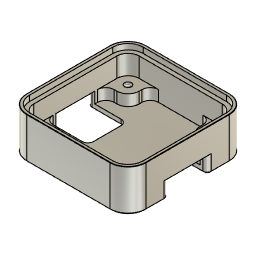
simplest_knob_case_tutorial (Autodesk Fusion 360 design; units mm, degrees)
Autodesk Fusion 360 part; units mm, degrees
sketch "sketch_for_main_body_shape" plane through (0, 0, 0) normal (0, 0, 1) x (1, 0, 0)
  line L0 (15, -18.5) -> (-15, -18.5) construction
  line L1 (-18.5, -15) -> (-18.5, 15) construction
  line L2 (-15, 18.5) -> (15, 18.5) construction
  line L3 (18.5, 15) -> (18.5, -15) construction
  line L4 (18.5, -18.5) -> (-18.5, 18.5) construction
  line L5 (-18.5, -18.5) -> (18.5, 18.5) construction
  arc A0 (-15, 18.5) -> (-18.5, 15) centre (-15, 15) ccw construction
  arc A1 (-18.5, -15) -> (-15, -18.5) centre (-15, -15) ccw construction
  arc A2 (15, -18.5) -> (18.5, -15) centre (15, -15) ccw construction
  arc A3 (18.5, 15) -> (15, 18.5) centre (15, 15) ccw construction
  arc A4 (19, 15) -> (15, 19) centre (15, 15) ccw
  line L6 (-15, 19) -> (15, 19)
  arc A5 (-15, 19) -> (-19, 15) centre (-15, 15) ccw
  line L7 (-19, -15) -> (-19, 15)
  arc A6 (-19, -15) -> (-15, -19) centre (-15, -15) ccw
  line L8 (15, -19) -> (-15, -19)
  arc A7 (15, -19) -> (19, -15) centre (15, -15) ccw
  line L9 (19, 15) -> (19, -15)
  arc A8 (21.5, 15) -> (15, 21.5) centre (15, 15) ccw
  line L10 (-15, 21.5) -> (15, 21.5)
  arc A9 (-15, 21.5) -> (-21.5, 15) centre (-15, 15) ccw
  line L11 (-21.5, -15) -> (-21.5, 15)
  arc A10 (-21.5, -15) -> (-15, -21.5) centre (-15, -15) ccw
  line L12 (15, -21.5) -> (-15, -21.5)
  arc A11 (15, -21.5) -> (21.5, -15) centre (15, -15) ccw
  line L13 (21.5, 15) -> (21.5, -15)
  circle A12 centre (-15, 15) radius 4
  line L14 (-11, 15) -> (-11, 19)
  line L15 (-15, 11) -> (-19, 11)
  circle A13 centre (15, 15) radius 4
  line L16 (11, 15) -> (11, 19)
  line L17 (15, 11) -> (19, 11)
  line L18 (-37.3211, 0) -> (37.3211, 0) construction
  line L19 (-11, -15) -> (-11, -19)
  circle A14 centre (-15, -15) radius 4
  line L20 (-15, -11) -> (-19, -11)
  circle A15 centre (15, -15) radius 4
  line L21 (15, -11) -> (19, -11)
  line L22 (11, -15) -> (11, -19)
  line L23 (-7.5, -7) -> (-21.5, -7)
  line L24 (-21.5, -7) -> (-21.5, 7)
  line L25 (-21.5, 7) -> (-7.5, 7)
  line L26 (-7.5, 7) -> (-7.5, -7)
  line L27 (21.5, -7) -> (7.5, -7)
  line L28 (7.5, -7) -> (7.5, 7)
  line L29 (7.5, 7) -> (21.5, 7)
  line L30 (21.5, 7) -> (21.5, -7)
  dimension "d6" = 37
  dimension "d7" = 37
  dimension "d8" = 3.5
  dimension "d9" = -0.5
  dimension "d10" = -3
  dimension "d21" = 14
  dimension "d22" = 14
  dimension "d23" = 14
  dimension "d24" = 14
  constraint horizontal L0
  constraint perpendicular L0 L1
  constraint parallel L0 L2
  constraint parallel L1 L3
  constraint coincident L4 origin
  constraint coincident L5 origin
  constraint coincident L4.end L2
  constraint coincident L4.end L1
  constraint tangent L2 A0
  constraint tangent L1 A0
  constraint coincident L5.start L1
  constraint coincident L5.start L0
  constraint tangent L1 A1
  constraint tangent L0 A1
  constraint equal A0 A1
  constraint coincident L4.start L0
  constraint coincident L4.start L3
  constraint tangent L0 A2
  constraint tangent L3 A2
  constraint equal A0 A2
  constraint coincident L5.end L3
  constraint coincident L5.end L2
  constraint tangent L3 A3
  constraint tangent L2 A3
  constraint equal A0 A3
  constraint concentric A0 A12
  constraint coincident L6.start A12
  constraint coincident A12 L14.start
  constraint coincident L6 L14.end
  constraint tangent A12 L14
  constraint vertical L14
  constraint coincident A12 L15.start
  constraint coincident L7 L15.end
  constraint tangent A12 L15
  constraint horizontal L15
  constraint concentric A3 A13
  constraint coincident A4.end A13
  constraint coincident A13 L16.start
  constraint coincident L6 L16.end
  constraint tangent A13 L16
  constraint perpendicular L6 L16
  constraint coincident A13 L17.start
  constraint coincident L9 L17.end
  constraint tangent A13 L17
  constraint perpendicular L9 L17
  constraint perpendicular L13 L18
  constraint midpoint origin L18
  constraint symmetric A12 L18 A14
  constraint symmetric L14.start L18 L19.start
  constraint symmetric L14.end L18 L19.end
  constraint symmetric L15.start L18 L20.start
  constraint symmetric L15.end L18 L20.end
  constraint symmetric A13 L18 A15
  constraint symmetric L16.start L18 L22.start
  constraint symmetric L16.end L18 L22.end
  constraint symmetric L17.start L18 L21.start
  constraint symmetric L17.end L18 L21.end
  constraint horizontal L23
  constraint vertical L24
  constraint horizontal L25
  constraint vertical L26
  constraint midpoint L11 L24
  constraint horizontal L27
  constraint vertical L28
  constraint horizontal L29
  constraint vertical L30
  constraint midpoint L13 L30
  measures "d6" distance of L4.end L5.end
  measures "d7" distance of L5.start L4.end
  measures "d8" radius of A0
  measures "d21" distance of L23.start L23.end
  measures "d22" distance of L23.start L25.end
  measures "d23" distance of L27.start L27.end
  measures "d24" distance of L27.start L29.end
extrude "Extrude1" add sketch "sketch_for_main_body_shape" along normal blind 2
extrude "Extrude2" add sketch "sketch_for_main_body_shape" along normal blind 15 contours A4 L6 A5 L7 L9 A8 L10 A9 L11 L13 A12 A13 L25 L29 | L9 L13 L27 L29 L30 | L7 A6 L8 A7 L9 L11 A10 L12 A11 L13 A14 A15 L23 L27 | L7 L11 L23 L24 L25
extrude "Extrude3" add sketch "sketch_for_main_body_shape" along normal blind 6 contours A4 A13 | L9 A13 L17 | L6 A13 L16 | L6 A12 L14 | A5 A12 | L9 A15 L21 | L7 A12 L15 | A7 A15 | L8 A15 L22 | L8 L19 A14 | L7 A14 L20 | A6 A14
sketch "sketch_for_holes" plane through (0, 0, 6) normal (0, 0, 1) x (-1, 0, 0)
  line L0 (11, -15) -> (11, -19)
  line L1 (11, -19) -> (15, -19)
  arc A0 (15, -19) -> (19, -15) centre (15, -15) ccw
  line L2 (19, -15) -> (19, -11)
  line L3 (19, -11) -> (15, -11)
  arc A1 (15, -11) -> (11, -15) centre (15, -15) ccw
  point P0 (-15, -15)
  point P1 (15, -15)
  point P2 (15, 15)
  point P3 (-15, 15)
hole "Hole1" at (-15, 15, 6) at (15, 15, 6) at (15, -15, 6) at (-15, -15, 6) direction (0, 0, -1) diameter 2.529 depth 4 tip angle 118
thread "Thread1" "ISO Metric profile 3.0 M3x0.5 6H"
extrude "Extrude4" cut sketch "sketch_for_main_body_shape" along normal blind 6 contours L9 L13 L27 L29 L30 | L9 L27 L28 L29 | L7 L23 L25 L26 | L7 L11 L23 L24 L25
sketch "sketch_for_rim" plane through (0, 0, 15) normal (0, 0, 1) x (-1, 0, 0)
  arc A0 (15, -19) -> (19, -15) centre (15, -15) ccw
  line L0 (15, -19) -> (-15, -19)
  arc A1 (-19, -15) -> (-15, -19) centre (-15, -15) ccw
  line L1 (-19, -15) -> (-19, 15)
  arc A2 (-15, 19) -> (-19, 15) centre (-15, 15) ccw
  line L2 (-15, 19) -> (15, 19)
  arc A3 (19, 15) -> (15, 19) centre (15, 15) ccw
  line L3 (19, 15) -> (19, -15)
  arc A4 (15, -21.5) -> (21.5, -15) centre (15, -15) ccw
  line L4 (21.5, -15) -> (21.5, 15)
  arc A5 (21.5, 15) -> (15, 21.5) centre (15, 15) ccw
  line L5 (15, 21.5) -> (-15, 21.5)
  arc A6 (-15, 21.5) -> (-21.5, 15) centre (-15, 15) ccw
  line L6 (-21.5, 15) -> (-21.5, -15)
  arc A7 (-21.5, -15) -> (-15, -21.5) centre (-15, -15) ccw
  line L7 (-15, -21.5) -> (15, -21.5)
  arc A8 (20.5, 15) -> (15, 20.5) centre (15, 15) ccw
  line L8 (-15, 20.5) -> (15, 20.5)
  arc A9 (-15, 20.5) -> (-20.5, 15) centre (-15, 15) ccw
  line L9 (-20.5, -15) -> (-20.5, 15)
  arc A10 (-20.5, -15) -> (-15, -20.5) centre (-15, -15) ccw
  line L10 (15, -20.5) -> (-15, -20.5)
  arc A11 (15, -20.5) -> (20.5, -15) centre (15, -15) ccw
  line L11 (20.5, 15) -> (20.5, -15)
  dimension "d27" = -1.5
extrude "Extrude5" cut sketch "sketch_for_rim" against normal blind 2 contours A8 L8 A9 L9 A10 L10 A11 L11
fillet "Fillet1" radius 3 8 edges at (11, -19, 4) (19, -11, 4) (19, 11, 4) (11, 19, 4) (-11, 19, 4) (-19, 11, 4) (-19, -11, 4) (-11, -19, 4)
fillet "Fillet2" radius 2 4 edges at (7.5, -7, 1) (7.5, 7, 1) (-7.5, 7, 1) (-7.5, -7, 1)
fillet "Fillet3" radius 1.5 4 edges at (-21.5, 7, 3) (-21.5, -7, 3) (21.5, -7, 3) (21.5, 7, 3)
chamfer "Chamfer1" distance 0.5 angle 45 24 edges at (0, -21.5, 0) (-19.5962, -19.5962, 0) (-21.5, -11.75, 0) (-21.0607, -7.4393, 0) (-14.75, -7, 0) (-8.0858, -6.4142, 0) (-7.5, 0, 0) (-8.0858, 6.4142, 0) (-14.75, 7, 0) (-21.0607, 7.4393, 0) (-21.5, 11.75, 0) (-19.5962, 19.5962, 0) (0, 21.5, 0) (19.5962, 19.5962, 0) (21.5, 11.75, 0) (21.0607, 7.4393, 0) (14.75, 7, 0) (8.0858, 6.4142, 0) (7.5, 0, 0) (8.0858, -6.4142, 0) (14.75, -7, 0) (21.0607, -7.4393, 0) (21.5, -11.75, 0) (19.5962, -19.5962, 0)
chamfer "Chamfer2" distance 0.1 angle 45 8 edges at (21.5, 0, 15) (19.5962, 19.5962, 15) (0, 21.5, 15) (-19.5962, 19.5962, 15) (-21.5, 0, 15) (-19.5962, -19.5962, 15) (0, -21.5, 15) (19.5962, -19.5962, 15)
equation "d21 = 11 mm + 3 mm"
named bodies: "enclosure_for_rotary_encoder_module"
